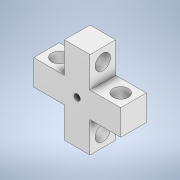
# Autodesk Inventor part: シリンダ先端パーツ
Saved by Autodesk Inventor 2021 (Build 250183000, 183)
## iProperties
Created: 2021-10-09
Part Number: シリンダ先端パーツ
Material: 一般
Document SubType Name: Modeling
Designer: ryusei
Density: 1 g/cm^3
Appearance: 滑らか - 白
Author: ryusei
Autodesk Inventor part; units mm, degrees
ref_plane "YZ Plane" through (0, 0, 0) normal (1, 0, 0) x (0, 1, 0)
ref_plane "XZ Plane" through (0, 0, 0) normal (0, 1, 0) x (-1, 0, 0)
ref_plane "XY Plane" through (0, 0, 0) normal (0, 0, 1) x (1, 0, 0)
sketch "スケッチ1" plane through (0, 0, 0) normal (0, 0, 1) x (1, 0, 0)
  line L0 (0, 0) -> (34, 0)
  line L1 (34, 0) -> (34, 34)
  line L2 (34, 34) -> (0, 34)
  line L3 (0, 34) -> (0, 0)
  dimension "d0" = 34
  dimension "d1" = 34
  constraints: 8 end point, 2 parallel, 1 horizontal, 1 perpendicular
  measures "d0" distance between parallel lines of L1 L3
  measures "d1" distance between parallel lines of L0 L2
extrude "押し出し1" add sketch "スケッチ1" along normal blind 10
sketch "スケッチ2" plane through (0, 0, 10) normal (0, 0, 1) x (1, 0, 0)
  line L0 (34, 34) -> (0, 34) projected
  line L1 (34, 34) -> (22, 34)
  line L2 (22, 34) -> (22, 22)
  line L3 (22, 22) -> (34, 22)
  line L4 (34, 22) -> (34, 34)
  point P0 (0, 0)
  point P1 (22, 34)
  dimension "d4" = 12
  dimension "d5" = 12
  constraints: 8 end point, 2 parallel, 1 horizontal, 1 perpendicular
  measures "d4" distance of L1.end L2.end
  measures "d5" distance of L2.end L3.end
extrude "押し出し2" cut sketch "スケッチ2" against normal blind 10
sketch "スケッチ3" plane through (0, 0, 10) normal (0, 0, 1) x (1, 0, 0)
  line L0 (0, 34) -> (12, 34)
  line L1 (12, 34) -> (12, 22)
  line L2 (12, 22) -> (0, 22)
  line L3 (0, 22) -> (0, 34)
  line L4 (0, 0) -> (34, 0) projected
  line L5 (0, 0) -> (12, 0)
  line L6 (12, 0) -> (12, 12)
  line L7 (12, 12) -> (0, 12)
  line L8 (0, 12) -> (0, 0)
  line L9 (34, 0) -> (22, 0)
  line L10 (22, 0) -> (22, 12)
  line L11 (22, 12) -> (34, 12)
  line L12 (34, 12) -> (34, 0)
  point P0 (22, 0)
  dimension "d8" = 12
  dimension "d9" = 12
  dimension "d10" = 12
  dimension "d11" = 12
  dimension "d12" = 12
  dimension "d13" = 12
  constraints: 24 end point, 6 parallel, 3 horizontal, 3 perpendicular
  measures "d8" distance of L1.end L2.end
  measures "d9" distance of L0.end L1.end
  measures "d10" distance of L6.end L7.end
  measures "d11" distance of L5.end L6.end
  measures "d12" distance of L9.end L10.end
  measures "d13" distance of L10.end L11.end
extrude "押し出し3" cut sketch "スケッチ3" against normal blind 10
sketch "スケッチ4" plane through (22, 22, 10) normal (1, 0, 0) x (0, 0, -1)
  line L0 (0, 12) -> (10, 12) projected
  line L1 (10, 12) -> (10, 0) projected
  line L2 (10, -10) -> (10, -22) projected
  line L3 (10, -22) -> (0, -22) projected
  point P0 (5, 7)
  point P1 (5, -17)
  dimension "d16" = 5
  dimension "d17" = 5
  dimension "d18" = 5
  dimension "d19" = 5
  measures "d16" distance from line of L0 point (5, 7)
  measures "d17" distance from line of L1 point (5, 7)
  measures "d18" distance from line of L2 point (5, -17)
  measures "d19" distance from line of L3 point (5, -17)
hole "穴1" at (22, 29, 5) at (22, 5, 5) direction (-1, 0, 0) diameter 6 end through all
sketch "スケッチ5" plane through (0, 22, 10) normal (0, 1, 0) x (1, 0, 0)
  line L0 (0, 10) -> (12, 10) projected
  line L1 (0, 0) -> (0, 10) projected
  line L2 (22, 10) -> (34, 10) projected
  line L3 (34, 10) -> (34, 0) projected
  point P0 (5, 5)
  point P1 (29, 5)
  dimension "d27" = 5
  dimension "d28" = 5
  dimension "d29" = 5
  dimension "d30" = 5
  measures "d27" distance from line of L0 point (5, 5)
  measures "d28" distance from line of L1 point (5, 5)
  measures "d29" distance from line of L2 point (29, 5)
  measures "d30" distance from line of L3 point (29, 5)
hole "穴2" at (5, 22, 5) at (29, 22, 5) direction (0, -1, 0) diameter 6 end through all
sketch "スケッチ6" plane through (0, 0, 10) normal (0, 0, 1) x (1, 0, 0)
  line L0 (34, 12) -> (34, 22) projected
  line L1 (22, 34) -> (12, 34) projected
  point P0 (0, 0)
  point P1 (17, 17)
  dimension "d38" = 17
  dimension "d39" = 17
  measures "d38" distance from line of L0 point (17, 17)
  measures "d39" distance from line of L1 point (17, 17)
hole "穴3" at (17, 17, 10) direction (0, 0, -1) diameter 2.459 end through all thread size "M3x0.5" class "6H" standard "ISO Metric profile"
